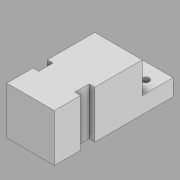
# Autodesk Inventor part: Box A01209499
Saved by Autodesk Inventor 2020 (Build 240168000, 168)
## iProperties
Created: 2019-10-15
Part Number: Box A01209499
Material: Genérico
Document SubType Name: Modeling
Designer: gerar
Density: 1 g/cm^3
Appearance: Valor por defecto
Author: gerar
Autodesk Inventor part; units mm, degrees
ref_plane "YZ Plane" through (0, 0, 0) normal (1, 0, 0) x (0, 1, 0)
ref_plane "XZ Plane" through (0, 0, 0) normal (0, 1, 0) x (-1, 0, 0)
ref_plane "XY Plane" through (0, 0, 0) normal (0, 0, 1) x (1, 0, 0)
sketch "Boceto1" plane through (0, 0, 0) normal (0, 1, 0) x (-1, 0, 0)
  line L0 (0, 0) -> (50.8, 0)
  line L1 (50.8, -93.98) -> (0, -93.98)
  line L2 (50.8, -27.94) -> (44.704, -27.94)
  line L3 (44.704, -27.94) -> (44.704, -43.18)
  line L4 (44.704, -43.18) -> (50.8, -43.18)
  line L5 (6.096, -27.94) -> (0, -27.94)
  line L6 (0, -43.18) -> (6.096, -43.18)
  line L7 (6.096, -43.18) -> (6.096, -27.94)
  line L8 (50.8, 0) -> (50.8, -27.94)
  line L9 (50.8, -43.18) -> (50.8, -93.98)
  line L10 (0, -93.98) -> (0, -43.18)
  line L11 (0, -27.94) -> (0, 0)
  dimension "d0" = 50.8
  dimension "d1" = 93.98
  dimension "d2" = 27.94
  dimension "d3" = 15.24
  dimension "d5" = 27.94
  dimension "d6" = 15.24
  constraints: 24 end point, 7 parallel, 3 horizontal, 3 perpendicular, 1 point on line
  measures "d0" distance of L1.start L1.end
  measures "d1" distance of L0.end L1.start
  measures "d2" distance between parallel lines of L0 L2
  measures "d3" distance between parallel lines of L2 L4
  measures "d5" distance between parallel lines of L0 L5
  measures "d6" distance between parallel lines of L6 L5
extrude "Extrusión1" add sketch "Boceto1" along normal blind 50.8
sketch "Boceto2" plane through (0, 0, 0) normal (0, 1, 0) x (-1, 0, 0)
  line L0 (0, -93.98) -> (50.8, -93.98) projected
  line L1 (0, -93.98) -> (50.8, -93.98)
  line L2 (50.8, -93.98) -> (50.8, -127)
  line L3 (50.8, -127) -> (0, -127)
  line L4 (0, -127) -> (0, -93.98)
  point P0 (0, 0)
  dimension "d10" = 50.8
  dimension "d11" = 33.02
  constraints: 8 end point, 2 parallel, 1 horizontal, 1 perpendicular
  measures "d10" distance of L2.end L3.end
  measures "d11" distance of L1.end L2.end
extrude "Extrusión2" add sketch "Boceto2" along normal blind 17.78
sketch "Boceto4" plane through (0, 50.8, -93.98) normal (0, 0, -1) x (-1, 0, 0)
  circle A0 centre (25.4, -25.4) radius 19.05 construction
  line L0 (0, -50.8) -> (50.8, -50.8) construction
  line L1 (0, -33.02) -> (0, 0) construction
  line L2 (6.35, -25.4) -> (15.875, -8.9022)
  line L3 (15.875, -8.9022) -> (34.925, -8.9022)
  line L4 (34.925, -8.9022) -> (44.45, -25.4)
  line L5 (44.45, -25.4) -> (34.925, -41.8978)
  line L6 (34.925, -41.8978) -> (15.875, -41.8978)
  line L7 (15.875, -41.8978) -> (6.35, -25.4)
  dimension "d19" = 38.1
  dimension "d20" = 25.4
  dimension "d21" = 25.4
  constraints: 12 end point, 1 coincident, 1 horizontal alignment, 15 other
  measures "d20" distance from line of L0 point (25.4, -25.4)
  measures "d21" distance from line of L1 point (25.4, -25.4)
extrude "Extrusión4" cut sketch "Boceto4" against normal blind 43.18
sketch "Boceto5" plane through (0, 0, 0) normal (0, -1, 0) x (1, 0, 0)
  line L0 (14.674, -110.236) -> (-74.6814, -110.236) construction
  line L1 (-12.7, -139.0037) -> (-12.7, -100.1648) construction
  line L2 (-38.1, -100.1648) -> (-38.1, -139.0037) construction
  line L3 (0, -43.18) -> (0, -127) projected
  line L4 (-50.8, -127) -> (-50.8, -43.18) projected
  line L5 (0, -127) -> (-50.8, -127) projected
  point P0 (0, 0)
  point P1 (-12.7, -110.236)
  point P2 (-38.1, -110.236)
  dimension "d24" = 12.7
  dimension "d25" = 12.7
  dimension "d26" = 25.4
  dimension "d27" = 16.764
  constraints: 6 end point, 4 point on line, 2 vertical, 1 horizontal
  measures "d24" distance between parallel lines of L1 L3
  measures "d25" distance between parallel lines of L2 L4
  measures "d26" distance between parallel lines of L2 L1
  measures "d27" distance between parallel lines of L0 L5
hole "Agujero1" at (-12.7, 0, -110.236) at (-38.1, 0, -110.236) direction (0, 1, 0) diameter 7.62 end through all counterbore diameter 9.652 counterbore depth 7.62
